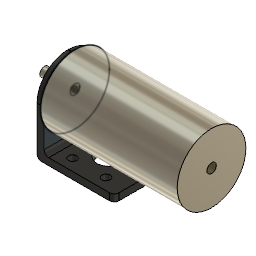
Motor bracket (Autodesk Fusion 360 design; units mm, degrees)
part number: 2026-02-05-14-44-17-191
Autodesk Fusion 360 part; units mm, degrees
sketch "Sketch1" plane through (0, 0, 0) normal (0, 0, 1) x (1, 0, 0)
  line L0 (0, 0) -> (30.8, 0)
  line L1 (32.8, 2) -> (32.8, 24.3)
  line L2 (30.8, 26.3) -> (0, 26.3)
  line L3 (0, 26.3) -> (0, 0)
  line L4 (3, 26.3) -> (3, 0)
  circle A0 centre (10.2, 21.4) radius 1.75
  circle A1 centre (24.4, 21.4) radius 1.75
  circle A2 centre (10.2, 4.9) radius 1.75
  circle A3 centre (24.4, 4.9) radius 1.75
  circle A4 centre (17.3, 13.15) radius 5
  line L5 (10.2, 4.9) -> (10.2, 21.4) construction
  line L6 (10.2, 21.4) -> (24.4, 21.4) construction
  line L7 (24.4, 21.4) -> (24.4, 4.9) construction
  line L8 (24.4, 4.9) -> (10.2, 4.9) construction
  arc A5 (32.8, 24.3) -> (30.8, 26.3) centre (30.8, 24.3) ccw
  arc A6 (30.8, 0) -> (32.8, 2) centre (30.8, 2) ccw
  line L9 (3, 13.15) -> (32.8, 13.15) construction
  point P0 (32.8, 0)
  point P1 (10.2, 13.15)
  point P2 (17.3, 21.4)
  point P3 (24.4, 13.15)
  point P4 (17.3, 4.9)
  dimension "d1" = 32.8
  dimension "d2" = 26.3
  dimension "d3" = 3
  dimension "d4" = 3.5
  dimension "d7" = 14.2
  dimension "d8" = -16.5
  dimension "d9" = 10
  dimension "d10" = 15.5
  dimension "d11" = 2
  constraint horizontal L0
  constraint vertical L1
  constraint horizontal L2
  constraint vertical L3
  constraint coincident L0.start L3.end
  constraint coincident L2 L4.start
  constraint coincident L0 L4.end
  constraint perpendicular L0 L4
  constraint coincident A2.centre L5.start
  constraint coincident A0.centre L5.end
  constraint coincident A1.centre L6.end
  constraint coincident A3.centre L7.end
  constraint midpoint L5 P1
  constraint midpoint L6 P2
  constraint midpoint L7 P3
  constraint midpoint L8 P4
  constraint horizontal A4.centre P1
  constraint vertical A4.centre P2
  constraint tangent L1 A5
  constraint tangent L2 A5
  constraint coincident P0 L0
  constraint coincident P0 L1
  constraint tangent L0 A6
  constraint tangent L1 A6
  constraint equal A5 A6
  constraint midpoint L4 L9.start
  constraint midpoint L1 L9.end
  constraint coincident A4.centre L9
  measures "d1" distance of L0.start P0
  measures "d2" distance of L0.start L2.end
  measures "d3" distance of L3 L4
  measures "d4" diameter of A0
  measures "d9" diameter of A4
  measures "d10" distance of L1 A4.centre
  measures "d11" radius of A5
extrude "Extrude1" add sketch "Sketch1" along normal blind 3 contours L0 L1 L2 L4 A5 A6 makes body 1
extrude "Extrude2" add sketch "Sketch1" along normal blind 33.7 contours L0 L2 L3 L4 bodies 1
fillet "Fillet1" radius 13.1 2 edges at (1.5, 0, 33.7) (1.5, 26.3, 33.7) on bodies 1
sketch "Sketch2" plane through (0, 0, 0) normal (-1, 0, 0) x (0, -1, 0)
  arc A0 (-13.2, 33.7) -> (-26.3, 20.6) centre (-13.2, 20.6) ccw
  line L0 (-26.3, 20.6) -> (-26.3, 0)
  line L1 (-26.3, 0) -> (0, 0)
  line L2 (0, 0) -> (0, 20.6)
  arc A1 (0, 20.6) -> (-13.1, 33.7) centre (-13.1, 20.6) ccw
  line L3 (-13.1, 33.7) -> (-13.2, 33.7)
  line L4 (-26.3, 20.6) -> (0, 20.6) construction
  circle A2 centre (-13.15, 20.6) radius 4
  circle A3 centre (-21.8, 20.6) radius 1.85
  line L5 (-13.15, 0) -> (-13.15, 33.7) construction
  circle A4 centre (-4.5, 20.6) radius 1.85
  point P0 (-13.15, 20.6)
  dimension "d18" = 8
  dimension "d19" = 3.7
  dimension "d20" = 8.65
  constraint coincident A0.end L0.start
  constraint coincident L2.end A1.start
  constraint midpoint L4 P0
  constraint coincident P0 A2.centre
  constraint coincident L4 A3.centre
  constraint midpoint L1 L5.start
  constraint midpoint L3 L5.end
  constraint symmetric A3 L5 A4
  measures "d18" diameter of A2
  measures "d19" diameter of A3
  measures "d20" distance of P0 A3.centre
extrude "Extrude3" cut sketch "Sketch2" against normal blind 6 contours A2 | A3 | A4 bodies 1
fillet "Fillet2" radius 2 2 edges at (3, 13.15, 3) (0, 13.15, 0) on bodies 1
sketch "Sketch3" plane through (3, 0, 0) normal (1, 0, 0) x (0, 1, 0)
  line L0 (0, 5) -> (26.3, 5)
  line L1 (26.3, 5) -> (26.3, 20.6)
  arc A0 (26.3, 20.6) -> (13.2, 33.7) centre (13.2, 20.6) ccw
  line L2 (13.2, 33.7) -> (13.1, 33.7)
  arc A1 (13.1, 33.7) -> (0, 20.6) centre (13.1, 20.6) ccw
  line L3 (0, 20.6) -> (0, 5)
  circle A2 centre (4.5, 20.6) radius 1.85
  circle A3 centre (13.15, 20.6) radius 4
  circle A4 centre (21.8, 20.6) radius 1.85
  circle A5 centre (13.15, 20.6) radius 14.6
  circle A6 centre (13.15, 20.6) radius 2
  dimension "d25" = 29.2
  dimension "d26" = 4
  constraint concentric A3 A5
  constraint concentric A5 A6
  measures "d25" diameter of A5
  measures "d26" diameter of A6
extrude "Extrude4" add sketch "Sketch3" along normal blind 58 contours L1 A0 L2 A1 L3 A5 | L1 A0 L2 A1 L3 A5 | A2 | A3 | A4 bodies 1
extrude "Extrude5" add sketch "Sketch3" against normal blind 13 separate body contours A6 makes body 2
equation "d7 = 17.7 mm - 3.5 mm"
equation "d8 = -( 20 mm - 3.5 mm )"
equation "d10 = 10.5 mm + 5 mm"
equation "d20 = 2.8 mm + ( ( 3.7 / 2 ) * 1 mm ) + ( ( 8 / 2 ) * 1 mm )"
